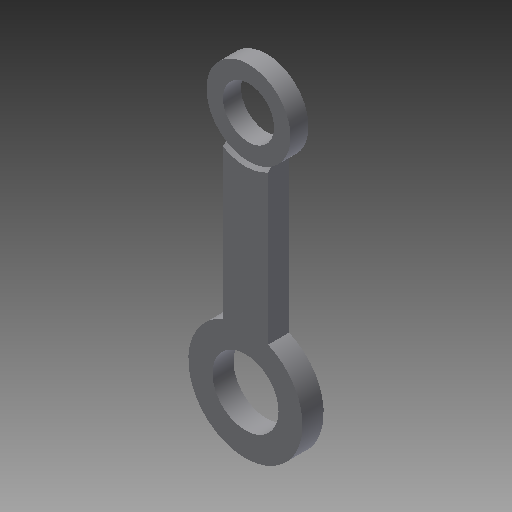
# Autodesk Inventor part: con rod
Saved by Autodesk Inventor 2017 SP1 (Build 210196100, 196)
## iProperties
Created: 2017-06-14
Part Number: con rod
Material: Generic
Document SubType Name: Modeling
Designer: RMcComber
Density: 1 g/cm^3
Appearance: Default
Author: RMcComber
Autodesk Inventor part; units mm, degrees
ref_plane "YZ Plane" through (0, 0, 0) normal (1, 0, 0) x (0, 1, 0)
ref_plane "XZ Plane" through (0, 0, 0) normal (0, 1, 0) x (-1, 0, 0)
ref_plane "XY Plane" through (0, 0, 0) normal (0, 0, 1) x (1, 0, 0)
sketch "Sketch1" plane through (0, 0, 0) normal (0, 0, 1) x (1, 0, 0)
  line L0 (0, 0) -> (0, 80) construction
  circle A0 centre (0, 0) radius 11
  circle A1 centre (0, 80) radius 8.5
  line L1 (7.5, 17.4571) -> (-7.5, 17.4571)
  line L2 (-7.5, 17.4571) -> (-7.5, 68.1784)
  line L3 (-7.5, 68.1784) -> (7.5, 68.1784)
  line L4 (7.5, 68.1784) -> (7.5, 17.4571)
  line L5 (7.5, 17.4571) -> (-7.5, 68.1784) construction
  line L6 (-7.5, 17.4571) -> (7.5, 68.1784) construction
  arc A2 (7.5, 68.1784) -> (-7.5, 68.1784) centre (0, 80) ccw
  arc A3 (-7.5, 17.4571) -> (7.5, 17.4571) centre (0, 0) ccw
  point P0 (0, 42.8177)
  point P1 (0, 42.8177)
  dimension "d0" = 22
  dimension "d1" = 17
  dimension "d2" = 80
  dimension "d3" = 5.5
  dimension "d4" = 8
  dimension "d5" = 15
  constraints: 14 end point, 4 centre point, 4 coincident, 4 point on circle, 3 midpoint, 2 parallel, 1 horizontal, 1 perpendicular, 1 point on line, 1 vertical
  measures "d0" diameter of A0
  measures "d1" diameter of A1
  measures "d2" distance of L0.start L0.end
  measures "d3" radial gap between concentric circles of A1 A2
  measures "d4" radial gap between concentric circles of A0 A3
  measures "d5" distance between parallel lines of L4 L2
extrude "Extrusion1" add sketch "Sketch1" along normal blind 7
sketch "Sketch2" plane through (0, 0, 7) normal (0, 0, 1) x (1, 0, 0)
  circle A0 centre (0, 80) radius 8.5 projected
  arc A1 (7.5, 68.1784) -> (-7.5, 68.1784) centre (0, 80) ccw projected
  circle A2 centre (0, 80) radius 14
  constraints: 1 coincident, 3 other
extrude "Extrusion2" cut sketch "Sketch2" against normal blind 1
chamfer "Chamfer1" distance 1 angle 45 1 edges at (0, 66, 7)
body "Solid1"
